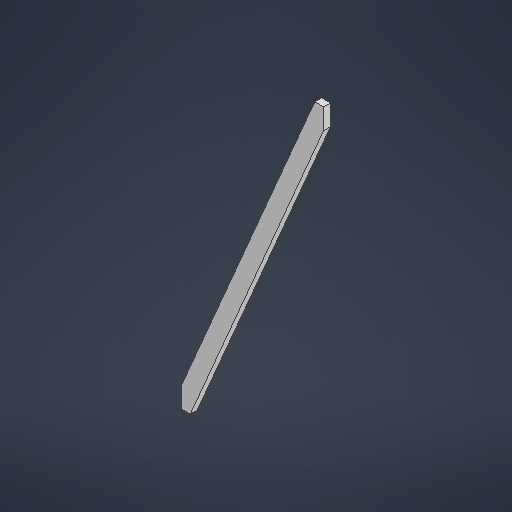
# Autodesk Inventor part: S_2x4x78.292
Saved by Autodesk Inventor 2026 (Build 300175000, 175)
## iProperties
Created: 2025-09-05
Part Number: S_2x4x78.292
Material: Generic
Document SubType Name: Modeling
Designer: trott
Density: 1 g/cm^3
Appearance: Default
Author: trott
Autodesk Inventor part; units mm, degrees
ref_plane "YZ Plane" through (0, 0, 0) normal (1, 0, 0) x (0, 1, 0)
ref_plane "XZ Plane" through (0, 0, 0) normal (0, 1, 0) x (-1, 0, 0)
ref_plane "XY Plane" through (0, 0, 0) normal (0, 0, 1) x (1, 0, 0)
sketch "Sketch1" plane through (0, 0, 0) normal (0, 0, 1) x (1, 0, 0)
  line L0 (0, 0) -> (781.05, 0)
  line L1 (0, 0) -> (0, 1828.8)
  line L2 (0, 1828.8) -> (781.05, 1828.8)
  line L3 (781.05, 1828.8) -> (781.05, 0)
  line L4 (0, 0) -> (781.05, 1828.8)
  line L5 (821.928, 1811.3417) -> (740.172, 1846.2583)
  line L6 (40.878, -17.4583) -> (-40.878, 17.4583)
  line L7 (740.172, 1846.2583) -> (-40.878, 17.4583)
  line L8 (40.878, -17.4583) -> (821.928, 1811.3417)
  point P0 (732.7159, 1828.8)
  point P1 (0, 113.1726)
  point P2 (48.3341, 0)
  point P3 (781.05, 1715.6274)
  dimension "d0" = 781.05
  dimension "d1" = 1828.8
  dimension "d2" = 88.9
  dimension "d3" = 88.9
  constraints: 18 end point, 3 perpendicular, 2 midpoint, 1 horizontal, 1 parallel, 1 vertical
  measures "d0" distance of L0.start L0.end
  measures "d1" distance of L0.start L1.end
  measures "d2" distance of L5.start L5.end
  measures "d3" distance of L6.start L6.end
extrude "Extrusion1" add sketch "Sketch1" along normal blind 38.1 contours L4 L3 L8 L0 | L1 L7 L2 L4
body "Solid1"
